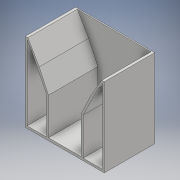
# Autodesk Inventor part: qzawsxedcfvgbhnjmk,l.
Saved by Autodesk Inventor 2017.3 (Build 213256000, 256)
## iProperties
Part Number: qzawsxedcfvgbhnjmk,l.
Material: Типовые
Document SubType Name: Modeling
Designer: ahmad
Density: 1 g/cm^3
Appearance: По умолчанию
Author: ahmad
Autodesk Inventor part; units mm, degrees
ref_plane "YZ Plane" through (0, 0, 0) normal (1, 0, 0) x (0, 1, 0)
ref_plane "XZ Plane" through (0, 0, 0) normal (0, 1, 0) x (-1, 0, 0)
ref_plane "XY Plane" through (0, 0, 0) normal (0, 0, 1) x (1, 0, 0)
sketch "Эскиз1" plane through (0, 0, 0) normal (0, 1, 0) x (-1, 0, 0)
  line L0 (-115, -115) -> (115, -115)
  line L1 (115, -115) -> (115, 115)
  line L2 (-115, 115) -> (-115, -115)
  line L3 (-115, -115) -> (115, 115) construction
  line L4 (115, -115) -> (-115, 115) construction
  line L5 (-107.5, -107.5) -> (107.5, -107.5)
  line L6 (107.5, -107.5) -> (107.5, 107.5)
  line L7 (-107.5, 107.5) -> (-107.5, -107.5)
  line L8 (-107.5, -107.5) -> (107.5, 107.5) construction
  line L9 (107.5, -107.5) -> (-107.5, 107.5) construction
  line L10 (107.5, 107.5) -> (107.5, 115)
  line L11 (-107.5, 107.5) -> (-107.5, 115)
  line L12 (115, 115) -> (107.5, 115)
  line L13 (-107.5, 115) -> (-115, 115)
  line L14 (107.5, 115) -> (74.5, 57.8423)
  line L15 (107.5, 115) -> (173.5, 115) construction
  line L16 (74.5, 57.8423) -> (47.5277, 0)
  line L17 (74.5, 57.8423) -> (138.3219, 57.8423) construction
  line L18 (47.5277, 0) -> (47.5277, -107.5)
  line L19 (-107.5, 115) -> (-74.5, 57.8423)
  line L20 (-107.5, 115) -> (-41.5, 115) construction
  line L21 (-74.5, 57.8423) -> (-47.5277, 0)
  line L22 (-74.5, 57.8423) -> (-10.6781, 57.8423) construction
  line L23 (-47.5277, 0) -> (-47.5277, -107.5)
  point P0 (0, 0)
  dimension "d0" = 230
  dimension "d1" = 230
  dimension "d4" = 66
  dimension "d5" = 120
  dimension "d6" = 115
  dimension "d7" = 66
  dimension "d8" = 60
  dimension "d9" = 65
  constraints: 48 end point, 6 horizontal, 5 perpendicular, 4 equal length, 4 midpoint, 4 parallel, 2 point on line, 2 vertical
  measures "d0" distance of L2.start L1.end
  measures "d1" distance of L1.end L0.end
  measures "d4" distance of L10.end L14.end
  measures "d5" angle of L14 L15
  measures "d6" angle of L16 L17
  measures "d7" distance of L11.end L19.end
  measures "d8" angle of L19 L20
  measures "d9" angle of L21 L22
extrude "Выдавливание1" add sketch "Эскиз1" along normal blind 150
sketch "Эскиз2" plane through (0, 150, 0) normal (0, 1, 0) x (1, 0, 0)
  line L0 (97.5879, -89.6233) -> (53.6439, -0.306)
  line L1 (53.6439, -0.306) -> (53.6439, 108.3759)
  line L2 (53.6439, 108.3759) -> (109.6776, 108.3759)
  line L3 (109.6776, 108.3759) -> (109.6776, -107.4647)
  line L4 (109.6776, -107.4647) -> (97.5879, -89.6233)
  line L5 (0, -179.4064) -> (0, 240.0482)
  line L6 (-97.5879, -89.6233) -> (-53.6439, -0.306)
  line L7 (-53.6439, -0.306) -> (-53.6439, 108.3759)
  line L8 (-53.6439, 108.3759) -> (-109.6776, 108.3759)
  line L9 (-109.6776, 108.3759) -> (-109.6776, -107.4647)
  line L10 (-109.6776, -107.4647) -> (-97.5879, -89.6233)
  point P0 (0, 0)
  constraints: 22 end point, 5 symmetric about line, 3 vertical, 1 perpendicular
extrude "Выдавливание2" cut sketch "Эскиз2" against normal blind 135161
sketch "Эскиз3" plane through (0, 150, 0) normal (0, 1, 0) x (1, 0, 0)
  line L0 (-107.5, -115) -> (-115, -115) projected
  line L1 (115, 115) -> (-115, 115)
  line L2 (-115, 115) -> (-115, -115)
  line L3 (-115, -115) -> (115, -115)
  line L4 (115, -115) -> (115, 115)
  line L5 (115, 115) -> (-115, -115) construction
  line L6 (-115, 115) -> (115, -115) construction
  point P0 (0, 0)
  constraints: 12 end point, 2 midpoint, 2 parallel, 1 horizontal, 1 perpendicular
extrude "Выдавливание3" add sketch "Эскиз3" against normal blind 3
sketch "Эскиз4" plane through (0, 0, 0) normal (0, -1, 0) x (1, 0, 0)
  line L0 (-115, -115) -> (115, -115) projected
  line L1 (115, 115) -> (-115, 115)
  line L2 (-115, 115) -> (-115, -115)
  line L3 (-115, -115) -> (115, -115)
  line L4 (115, -115) -> (115, 115)
  line L5 (115, 115) -> (-115, -115) construction
  line L6 (-115, 115) -> (115, -115) construction
  point P0 (0, 0)
  dimension "d16" = 230
  dimension "d17" = 230
  constraints: 12 end point, 2 midpoint, 2 parallel, 1 horizontal, 1 perpendicular
  measures "d16" distance of L3.end L0.start
  measures "d17" distance of L0.start L1.end
extrude "Выдавливание4" cut sketch "Эскиз4" against normal blind 3
